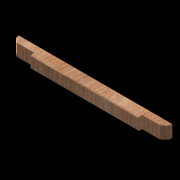
# Autodesk Inventor part: DNW_CON
Saved by Autodesk Inventor 2016 (Build 200138000, 138)
## iProperties
Created: 2017-08-22
Part Number: DNW_CON
Material: Wood (Birch)
Document SubType Name: Modeling
Designer: ludwi
Density: 0.55 g/cm^3
Appearance: Birch - Natural Polished
Author: ludwi
Autodesk Inventor part; units mm, degrees
ref_plane "YZ Plane" through (0, 0, 0) normal (1, 0, 0) x (0, 1, 0)
ref_plane "XZ Plane" through (0, 0, 0) normal (0, 1, 0) x (-1, 0, 0)
ref_plane "XY Plane" through (0, 0, 0) normal (0, 0, 1) x (1, 0, 0)
sketch "Sketch1" plane through (0, 0, 0) normal (0, 0, 1) x (1, 0, 0)
  line L0 (-357.1541, -65.4988) -> (-437.5068, -65.4988) construction
  line L1 (-357.1541, -65.4988) -> (-357.1541, -57.4988) construction
  line L2 (-357.1541, -57.4988) -> (-403.5317, -57.4988) construction
  line L3 (-415.2682, -47.6507) -> (-403.5317, -57.4988) construction
  line L4 (-415.2682, -47.6507) -> (-435.2333, 65.5771) construction
  line L5 (-431.1016, 70.5012) -> (-435.2333, 65.5771) construction
  line L6 (-431.1016, 70.5012) -> (-418.2505, 70.5012) construction
  line L7 (-418.2505, 70.5012) -> (-418.2505, 78.5012) construction
  line L8 (-518.2505, 78.5012) -> (-418.2505, 78.5012) construction
  line L9 (-518.2505, 78.5012) -> (-518.2505, 75.5012) construction
  line L10 (-518.2505, 75.5012) -> (-467.3689, 75.5012) construction
  line L11 (-461.5006, 70.5771) -> (-467.3689, 75.5012) construction
  line L12 (-461.5006, 70.5771) -> (-437.5068, -65.4988) construction
  line L13 (4.0058, -65.4988) -> (-76.3469, -65.4988) construction
  line L14 (4.0058, -65.4988) -> (27.9996, 70.5771) construction
  line L15 (33.8679, 75.5012) -> (27.9996, 70.5771) construction
  line L16 (33.8679, 75.5012) -> (84.7495, 75.5012) construction
  line L17 (84.7495, 75.5012) -> (84.7495, 78.5012) construction
  line L18 (-15.2505, 78.5012) -> (84.7495, 78.5012) construction
  line L19 (-15.2505, 78.5012) -> (-15.2505, 70.5012) construction
  line L20 (-15.2505, 70.5012) -> (-2.3994, 70.5012) construction
  line L21 (1.7323, 65.5771) -> (-2.3994, 70.5012) construction
  line L22 (1.7323, 65.5771) -> (-18.2328, -47.6507) construction
  line L23 (-29.9693, -57.4988) -> (-18.2328, -47.6507) construction
  line L24 (-29.9693, -57.4988) -> (-76.3469, -57.4988) construction
  line L25 (-76.3469, -57.4988) -> (-76.3469, -65.4988) construction
  line L26 (-357.1541, -67.4988) -> (-357.1541, -65.4988) construction
  line L27 (-357.1541, -65.4988) -> (-437.5068, -65.4988) construction
  line L28 (-437.5068, -65.4988) -> (-437.1541, -67.4988) construction
  line L29 (-437.1541, -67.4988) -> (-357.1541, -67.4988) construction
  line L30 (3.6531, -67.4988) -> (4.0058, -65.4988) construction
  line L31 (4.0058, -65.4988) -> (-76.3469, -65.4988) construction
  line L32 (-76.3469, -65.4988) -> (-76.3469, -67.4988) construction
  line L33 (-76.3469, -67.4988) -> (3.6531, -67.4988) construction
  line L34 (-416.865, -38.5948) -> (-16.636, -38.5948)
  line L35 (-16.636, -38.5948) -> (-18.2328, -47.6507)
  line L36 (-18.2328, -47.6507) -> (-29.9693, -57.4988)
  line L37 (-29.9693, -57.4988) -> (-76.3469, -57.4988)
  line L38 (-76.3469, -57.4988) -> (-76.3469, -67.4988)
  line L39 (-76.3469, -67.4988) -> (-357.1541, -67.4988)
  line L40 (-357.1541, -67.4988) -> (-357.1541, -57.4988)
  line L41 (-357.1541, -57.4988) -> (-403.5317, -57.4988)
  line L42 (-403.5317, -57.4988) -> (-415.2682, -47.6507)
  line L43 (-415.2682, -47.6507) -> (-416.865, -38.5948)
  constraints: 20 end point, 5 collinear, 3 perpendicular, 3 point on line, 1 horizontal
extrude "Extrusion1" add sketch "Sketch1" against normal blind 32
sketch "Sketch2" plane through (0, 0, 0) normal (0, 0, 1) x (1, 0, 0)
  line L0 (3.6531, -67.4988) -> (4.0058, -65.4988) projected
  line L1 (4.0058, -65.4988) -> (-76.3469, -65.4988) projected
  line L2 (-76.3469, -65.4988) -> (-76.3469, -67.4988) projected
  line L3 (-76.3469, -67.4988) -> (3.6531, -67.4988) projected
  line L4 (4.0058, -65.4988) -> (-76.3469, -65.4988) projected
  line L5 (4.0058, -65.4988) -> (27.118, 65.5771) projected
  line L6 (-15.2505, 78.5012) -> (-15.2505, 72.5012) projected
  line L7 (1.7323, 65.5771) -> (-18.5801, -49.6204) projected
  line L8 (-76.3469, -59.4988) -> (-76.3469, -65.4988) projected
  line L9 (-357.1541, -65.4988) -> (-437.5068, -65.4988) projected
  line L10 (-357.1541, -65.4988) -> (-357.1541, -59.4988) projected
  line L11 (-414.9209, -49.6204) -> (-435.2333, 65.5771) projected
  line L12 (-418.2505, 72.5012) -> (-418.2505, 78.5012) projected
  line L13 (-460.619, 65.5771) -> (-437.5068, -65.4988) projected
  line L14 (-357.1541, -67.4988) -> (-357.1541, -65.4988) projected
  line L15 (-357.1541, -65.4988) -> (-437.5068, -65.4988) projected
  line L16 (-437.5068, -65.4988) -> (-437.1541, -67.4988) projected
  line L17 (-437.1541, -67.4988) -> (-357.1541, -67.4988) projected
  line L18 (-357.1541, -57.4988) -> (-76.3469, -57.4988)
  line L19 (-76.3469, -57.4988) -> (-76.3469, -67.4988)
  line L20 (-76.3469, -67.4988) -> (-357.1541, -67.4988)
  line L21 (-357.1541, -67.4988) -> (-357.1541, -57.4988)
  line L22 (1.7323, 65.5771) -> (-4.0776, 72.5012) projected
  line L23 (-429.4234, 72.5012) -> (-435.2333, 65.5771) projected
  line L24 (35.3697, 72.5012) -> (27.118, 65.5771) projected
  line L25 (84.7495, 72.5012) -> (84.7495, 78.5012) projected
  line L26 (-518.2505, 78.5012) -> (-518.2505, 72.5012) projected
  line L27 (-460.619, 65.5771) -> (-468.8707, 72.5012) projected
  line L28 (-15.2505, 78.5012) -> (84.7495, 78.5012) projected
  line L29 (-518.2505, 78.5012) -> (-418.2505, 78.5012) projected
  line L30 (-76.3469, -59.4988) -> (-30.3528, -59.4988) projected
  line L31 (84.7495, 72.5012) -> (35.3697, 72.5012) projected
  line L32 (-4.0776, 72.5012) -> (-15.2505, 72.5012) projected
  line L33 (-30.3528, -59.4988) -> (-18.5801, -49.6204) projected
  line L34 (-414.9209, -49.6204) -> (-403.1482, -59.4988) projected
  line L35 (-418.2505, 72.5012) -> (-429.4234, 72.5012) projected
  line L36 (-468.8707, 72.5012) -> (-518.2505, 72.5012) projected
  line L37 (-403.1482, -59.4988) -> (-357.1541, -59.4988) projected
  point P0 (0, 0)
  constraints: 8 end point, 2 parallel, 1 horizontal, 1 perpendicular
extrude "Extrusion2" add sketch "Sketch2" against normal up to surface (32 mm away) contours L20 L14 L10 L21 L18 L19 L8 L2
chamfer "Chamfer1" distance 2 angle 45 2 edges at (-216.7505, -67.4988, -32) (-216.7505, -67.4988, 0)
body "Solid1"
